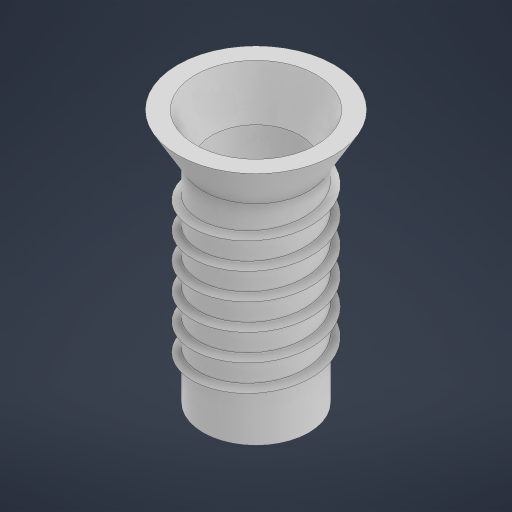
# Autodesk Inventor part: Oxy_B
Saved by Autodesk Inventor 2024.1 (Build 281209000, 209)
## iProperties
Created: 2024-08-16
Part Number: Oxy_B
Material: Generic
Document SubType Name: Modeling
Designer: Tim Jäger
Density: 1 g/cm^3
Appearance: Default
Author: Tim Jäger
## iProperties of the stored document Oxy_B_3DPrint.ipt
Created: 2024-08-17
Part Number: Oxy_B_3DPrint
Material: Generic
Document SubType Name: Modeling
Designer: Tim Jäger
Density: 1 g/cm^3
Appearance: Default
Author: Tim Jäger
Autodesk Inventor part; units mm, degrees
ref_plane "YZ Plane" through (0, 0, 0) normal (1, 0, 0) x (0, 1, 0)
ref_plane "XZ Plane" through (0, 0, 0) normal (0, 1, 0) x (-1, 0, 0)
ref_plane "XY Plane" through (0, 0, 0) normal (0, 0, 1) x (1, 0, 0)
sketch "Sketch1" plane through (0, 0, 0) normal (0, 0, 1) x (1, 0, 0)
  line L0 (8, 0) -> (8, 2.5)
  line L1 (8, 2.5) -> (10, 2.5)
  line L2 (10, 2.5) -> (10, 47.5)
  line L3 (10, 47.5) -> (12, 47.5)
  line L4 (12, 47.5) -> (12, 0)
  line L5 (12, 0) -> (8, 0)
  line L6 (0, -9.5) -> (0, 57) projected
  point P0 (0, 0)
  dimension "d0" = 2.5
  dimension "d1" = 12
  dimension "d2" = 8
  dimension "d3" = 2
  dimension "d4" = 47.5
  constraints: 12 end point, 5 perpendicular, 1 horizontal alignment, 1 vertical
  measures "d0" distance of L0.start L0.end
  measures "d1" distance from line of point (0, 0) L4
  measures "d2" distance from line of point (0, 0) L0
  measures "d3" distance between parallel lines of L4 L2
  measures "d4" distance of L3.end L4.end
revolve "Revolution1" add sketch "Sketch1" angle 360 about axis through (0, -10, 0) along (0, 1, 0)
sketch "Sketch2" plane through (0, 0, 0) normal (1, 0, 0) x (0, 1, 0)
  line L0 (0, -12) -> (47.5, -12) projected
  line L1 (44.5, -12) -> (43.6, -13.5588)
  line L2 (43.6, -13.5588) -> (42.7, -12)
  point P0 (0, 0)
  dimension "d6" = 60
  dimension "d7" = 1.8
  dimension "d8" = 3
  constraints: 4 end point, 2 point on line, 1 coincident, 1 equal length
  measures "d6" angle of L1 L2
  measures "d7" distance of L1.start L2.end
  measures "d8" distance of L1.start point (47.5, -12)
coil "Coil1" sketch "Sketch2" operation add axis through (0, -10, 0) along (0, -1, 0) pitch 6 turns 6 hand right
sketch "Sketch3" plane through (0, 0, 0) normal (1, 0, 0) x (0, 1, 0)
  line L0 (47.5, -10) -> (47.5, 10) projected
  line L1 (47.5, -12) -> (47.5, 12) projected
  line L2 (47.5, -10) -> (47.5, -12)
  line L3 (47.5, -12) -> (57.5, -17.7735)
  line L4 (57.5, -17.7735) -> (57.5, -13.7735)
  line L5 (57.5, -13.7735) -> (47.5, -10)
  line L6 (-11.5, 0) -> (69, 0) projected
  point P0 (0, 0)
  dimension "d17" = 120
  dimension "d18" = 4
  dimension "d19" = 10
  constraints: 8 end point, 1 parallel, 1 vertical
  measures "d17" angle of L1 L3
  measures "d18" distance of L3.end L4.end
  measures "d19" distance from line of L1.start L4
revolve "Revolution2" add sketch "Sketch3" angle 360 about axis through (0, -10, 0) along (0, 1, 0)
body "Solid1"
